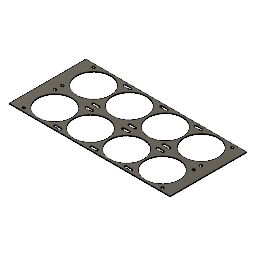
Corsair_1000D_120mm_x_8_fantray_extruded_v0 (Autodesk Fusion 360 design; units mm, degrees)
Autodesk Fusion 360 part; units mm, degrees
sketch "Sketch1" plane through (0, 0, 0) normal (0, 0, 1) x (1, 0, 0)
  line L0 (0, 0) -> (540, 0)
  line L1 (540, 0) -> (540, 258.064)
  line L2 (540, 258.064) -> (0, 258.064)
  line L3 (0, 258.064) -> (0, 0)
  circle A0 centre (89.662, 194.056) radius 56.642
  circle A1 centre (209.446, 194.056) radius 56.642
  line L4 (270, 258.064) -> (270, 0)
  line L5 (0, 129.032) -> (540, 129.032)
  circle A2 centre (450.3379, 194.056) radius 56.642
  circle A3 centre (330.5539, 194.056) radius 56.642
  circle A4 centre (89.662, 64.008) radius 56.642
  circle A5 centre (209.446, 64.008) radius 56.642
  circle A6 centre (330.5539, 64.008) radius 56.642
  circle A7 centre (450.3379, 64.008) radius 56.642
  line L6 (35.814, 249.428) -> (39.37, 249.428)
  line L7 (41.91, 246.888) -> (41.91, 245.11)
  line L8 (39.37, 242.57) -> (35.814, 242.57)
  line L9 (33.274, 245.11) -> (33.274, 246.888)
  arc A8 (35.814, 249.428) -> (33.274, 246.888) centre (35.814, 246.888) ccw
  arc A9 (33.274, 245.11) -> (35.814, 242.57) centre (35.814, 245.11) ccw
  arc A10 (39.37, 242.57) -> (41.91, 245.11) centre (39.37, 245.11) ccw
  arc A11 (41.91, 246.888) -> (39.37, 249.428) centre (39.37, 246.888) ccw
  line L10 (33.274, 140.208) -> (33.274, 141.986)
  arc A12 (33.274, 140.208) -> (35.814, 137.668) centre (35.814, 140.208) ccw
  line L11 (35.814, 144.526) -> (39.37, 144.526)
  arc A13 (35.814, 144.526) -> (33.274, 141.986) centre (35.814, 141.986) ccw
  line L12 (39.37, 137.668) -> (35.814, 137.668)
  line L13 (41.91, 141.986) -> (41.91, 140.208)
  arc A14 (39.37, 137.668) -> (41.91, 140.208) centre (39.37, 140.208) ccw
  arc A15 (41.91, 141.986) -> (39.37, 144.526) centre (39.37, 141.986) ccw
  line L14 (500.6299, 242.57) -> (504.1859, 242.57)
  line L15 (498.0899, 246.888) -> (498.0899, 245.11)
  arc A16 (506.7259, 246.888) -> (504.1859, 249.428) centre (504.1859, 246.888) ccw
  arc A17 (504.1859, 242.57) -> (506.7259, 245.11) centre (504.1859, 245.11) ccw
  arc A18 (498.0899, 245.11) -> (500.6299, 242.57) centre (500.6299, 245.11) ccw
  arc A19 (500.6299, 249.428) -> (498.0899, 246.888) centre (500.6299, 246.888) ccw
  line L16 (504.1859, 249.428) -> (500.6299, 249.428)
  line L17 (506.7259, 245.11) -> (506.7259, 246.888)
  arc A20 (39.37, 8.636) -> (41.91, 11.176) centre (39.37, 11.176) ccw
  arc A21 (35.814, 15.494) -> (33.274, 12.954) centre (35.814, 12.954) ccw
  line L18 (39.37, 15.494) -> (35.814, 15.494)
  arc A22 (33.274, 11.176) -> (35.814, 8.636) centre (35.814, 11.176) ccw
  line L19 (35.814, 8.636) -> (39.37, 8.636)
  line L20 (41.91, 11.176) -> (41.91, 12.954)
  arc A23 (41.91, 12.954) -> (39.37, 15.494) centre (39.37, 12.954) ccw
  line L21 (33.274, 12.954) -> (33.274, 11.176)
  arc A24 (35.814, 120.396) -> (33.274, 117.856) centre (35.814, 117.856) ccw
  line L22 (39.37, 120.396) -> (35.814, 120.396)
  line L23 (35.814, 113.538) -> (39.37, 113.538)
  line L24 (33.274, 117.856) -> (33.274, 116.078)
  arc A25 (39.37, 113.538) -> (41.91, 116.078) centre (39.37, 116.078) ccw
  arc A26 (33.274, 116.078) -> (35.814, 113.538) centre (35.814, 116.078) ccw
  arc A27 (41.91, 117.856) -> (39.37, 120.396) centre (39.37, 117.856) ccw
  line L25 (41.91, 116.078) -> (41.91, 117.856)
  line L26 (141.224, 249.428) -> (161.544, 249.428)
  line L27 (164.084, 246.888) -> (164.084, 245.11)
  line L28 (161.544, 242.57) -> (141.224, 242.57)
  line L29 (138.684, 245.11) -> (138.684, 246.888)
  arc A28 (138.684, 245.11) -> (141.224, 242.57) centre (141.224, 245.11) ccw
  arc A29 (141.224, 249.428) -> (138.684, 246.888) centre (141.224, 246.888) ccw
  arc A30 (161.544, 242.57) -> (164.084, 245.11) centre (161.544, 245.11) ccw
  arc A31 (164.084, 246.888) -> (161.544, 249.428) centre (161.544, 246.888) ccw
  line L30 (283.944, 242.57) -> (263.624, 242.57)
  line L31 (261.084, 245.11) -> (261.084, 246.888)
  line L32 (263.624, 249.428) -> (283.944, 249.428)
  arc A32 (286.484, 246.888) -> (283.944, 249.428) centre (283.944, 246.888) ccw
  line L33 (286.484, 246.888) -> (286.484, 245.11)
  arc A33 (283.944, 242.57) -> (286.484, 245.11) centre (283.944, 245.11) ccw
  arc A34 (261.084, 245.11) -> (263.624, 242.57) centre (263.624, 245.11) ccw
  arc A35 (263.624, 249.428) -> (261.084, 246.888) centre (263.624, 246.888) ccw
  arc A36 (138.684, 245.11) -> (141.224, 242.57) centre (141.224, 245.11) ccw
  arc A37 (141.224, 249.428) -> (138.684, 246.888) centre (141.224, 246.888) ccw
  line L34 (164.084, 246.888) -> (164.084, 245.11)
  arc A38 (161.544, 242.57) -> (164.084, 245.11) centre (161.544, 245.11) ccw
  line L35 (138.684, 245.11) -> (138.684, 246.888)
  arc A39 (164.084, 246.888) -> (161.544, 249.428) centre (161.544, 246.888) ccw
  line L36 (141.224, 249.428) -> (161.544, 249.428)
  line L37 (161.544, 242.57) -> (141.224, 242.57)
  line L38 (138.684, 138.852) -> (138.684, 140.63)
  line L39 (164.084, 140.63) -> (164.084, 138.852)
  line L40 (141.224, 143.17) -> (161.544, 143.17)
  arc A40 (164.084, 140.63) -> (161.544, 143.17) centre (161.544, 140.63) ccw
  arc A41 (138.684, 138.852) -> (141.224, 136.312) centre (141.224, 138.852) ccw
  line L41 (161.544, 136.312) -> (141.224, 136.312)
  arc A42 (141.224, 143.17) -> (138.684, 140.63) centre (141.224, 140.63) ccw
  arc A43 (161.544, 136.312) -> (164.084, 138.852) centre (161.544, 138.852) ccw
  arc A44 (261.084, 138.852) -> (263.624, 136.312) centre (263.624, 138.852) ccw
  line L42 (261.084, 138.852) -> (261.084, 140.63)
  line L43 (283.944, 136.312) -> (263.624, 136.312)
  arc A45 (283.944, 136.312) -> (286.484, 138.852) centre (283.944, 138.852) ccw
  arc A46 (263.624, 143.17) -> (261.084, 140.63) centre (263.624, 140.63) ccw
  line L44 (286.484, 140.63) -> (286.484, 138.852)
  arc A47 (286.484, 140.63) -> (283.944, 143.17) centre (283.944, 140.63) ccw
  line L45 (263.624, 143.17) -> (283.944, 143.17)
  line L46 (378.4559, 136.312) -> (398.7759, 136.312)
  arc A48 (375.9159, 138.852) -> (378.4559, 136.312) centre (378.4559, 138.852) ccw
  arc A49 (378.4559, 143.17) -> (375.9159, 140.63) centre (378.4559, 140.63) ccw
  arc A50 (398.7759, 136.312) -> (401.3159, 138.852) centre (398.7759, 138.852) ccw
  line L47 (398.7759, 143.17) -> (378.4559, 143.17)
  arc A51 (401.3159, 140.63) -> (398.7759, 143.17) centre (398.7759, 140.63) ccw
  line L48 (375.9159, 140.63) -> (375.9159, 138.852)
  line L49 (401.3159, 138.852) -> (401.3159, 140.63)
  line L50 (375.9159, 246.888) -> (375.9159, 245.11)
  line L51 (401.3159, 245.11) -> (401.3159, 246.888)
  line L52 (378.4559, 242.57) -> (398.7759, 242.57)
  arc A52 (398.7759, 242.57) -> (401.3159, 245.11) centre (398.7759, 245.11) ccw
  line L53 (398.7759, 249.428) -> (378.4559, 249.428)
  arc A53 (375.9159, 245.11) -> (378.4559, 242.57) centre (378.4559, 245.11) ccw
  line L54 (375.9159, 246.888) -> (375.9159, 245.11)
  arc A54 (401.3159, 246.888) -> (398.7759, 249.428) centre (398.7759, 246.888) ccw
  arc A55 (378.4559, 249.428) -> (375.9159, 246.888) centre (378.4559, 246.888) ccw
  arc A56 (375.9159, 245.11) -> (378.4559, 242.57) centre (378.4559, 245.11) ccw
  arc A57 (378.4559, 249.428) -> (375.9159, 246.888) centre (378.4559, 246.888) ccw
  line L55 (378.4559, 242.57) -> (398.7759, 242.57)
  arc A58 (398.7759, 242.57) -> (401.3159, 245.11) centre (398.7759, 245.11) ccw
  arc A59 (401.3159, 246.888) -> (398.7759, 249.428) centre (398.7759, 246.888) ccw
  line L56 (398.7759, 249.428) -> (378.4559, 249.428)
  line L57 (401.3159, 245.11) -> (401.3159, 246.888)
  arc A60 (398.7759, 8.636) -> (401.3159, 11.176) centre (398.7759, 11.176) ccw
  arc A61 (375.9159, 11.176) -> (378.4559, 8.636) centre (378.4559, 11.176) ccw
  line L58 (401.3159, 12.954) -> (401.3159, 11.176)
  line L59 (398.7759, 8.636) -> (378.4559, 8.636)
  arc A62 (401.3159, 12.954) -> (398.7759, 15.494) centre (398.7759, 12.954) ccw
  arc A63 (378.4559, 15.494) -> (375.9159, 12.954) centre (378.4559, 12.954) ccw
  line L60 (401.3159, 12.954) -> (401.3159, 11.176)
  arc A64 (378.4559, 15.494) -> (375.9159, 12.954) centre (378.4559, 12.954) ccw
  line L61 (398.7759, 8.636) -> (378.4559, 8.636)
  line L62 (375.9159, 11.176) -> (375.9159, 12.954)
  line L63 (375.9159, 11.176) -> (375.9159, 12.954)
  arc A65 (401.3159, 12.954) -> (398.7759, 15.494) centre (398.7759, 12.954) ccw
  arc A66 (398.7759, 8.636) -> (401.3159, 11.176) centre (398.7759, 11.176) ccw
  arc A67 (375.9159, 11.176) -> (378.4559, 8.636) centre (378.4559, 11.176) ccw
  line L64 (378.4559, 15.494) -> (398.7759, 15.494)
  line L65 (378.4559, 15.494) -> (398.7759, 15.494)
  line L66 (401.3159, 119.212) -> (401.3159, 117.434)
  arc A68 (378.4559, 121.752) -> (375.9159, 119.212) centre (378.4559, 119.212) ccw
  line L67 (398.7759, 114.894) -> (378.4559, 114.894)
  arc A69 (398.7759, 114.894) -> (401.3159, 117.434) centre (398.7759, 117.434) ccw
  arc A70 (375.9159, 117.434) -> (378.4559, 114.894) centre (378.4559, 117.434) ccw
  line L68 (378.4559, 121.752) -> (398.7759, 121.752)
  arc A71 (401.3159, 119.212) -> (398.7759, 121.752) centre (398.7759, 119.212) ccw
  line L69 (375.9159, 117.434) -> (375.9159, 119.212)
  line L70 (141.224, 114.894) -> (161.544, 114.894)
  arc A72 (161.544, 114.894) -> (164.084, 117.434) centre (161.544, 117.434) ccw
  line L71 (138.684, 119.212) -> (138.684, 117.434)
  arc A73 (141.224, 121.752) -> (138.684, 119.212) centre (141.224, 119.212) ccw
  arc A74 (164.084, 119.212) -> (161.544, 121.752) centre (161.544, 119.212) ccw
  line L72 (161.544, 121.752) -> (141.224, 121.752)
  arc A75 (138.684, 117.434) -> (141.224, 114.894) centre (141.224, 117.434) ccw
  line L73 (164.084, 117.434) -> (164.084, 119.212)
  line L74 (141.224, 8.636) -> (161.544, 8.636)
  line L75 (141.224, 8.636) -> (161.544, 8.636)
  line L76 (161.544, 15.494) -> (141.224, 15.494)
  line L77 (138.684, 12.954) -> (138.684, 11.176)
  line L78 (138.684, 12.954) -> (138.684, 11.176)
  line L79 (164.084, 11.176) -> (164.084, 12.954)
  arc A76 (141.224, 15.494) -> (138.684, 12.954) centre (141.224, 12.954) ccw
  arc A77 (161.544, 8.636) -> (164.084, 11.176) centre (161.544, 11.176) ccw
  arc A78 (161.544, 8.636) -> (164.084, 11.176) centre (161.544, 11.176) ccw
  arc A79 (138.684, 11.176) -> (141.224, 8.636) centre (141.224, 11.176) ccw
  line L80 (161.544, 15.494) -> (141.224, 15.494)
  arc A80 (141.224, 15.494) -> (138.684, 12.954) centre (141.224, 12.954) ccw
  arc A81 (164.084, 12.954) -> (161.544, 15.494) centre (161.544, 12.954) ccw
  line L81 (164.084, 11.176) -> (164.084, 12.954)
  arc A82 (164.084, 12.954) -> (161.544, 15.494) centre (161.544, 12.954) ccw
  arc A83 (138.684, 11.176) -> (141.224, 8.636) centre (141.224, 11.176) ccw
  arc A84 (286.484, 119.212) -> (283.944, 121.752) centre (283.944, 119.212) ccw
  arc A85 (263.624, 121.752) -> (261.084, 119.212) centre (263.624, 119.212) ccw
  line L82 (263.624, 114.894) -> (283.944, 114.894)
  arc A86 (283.944, 114.894) -> (286.484, 117.434) centre (283.944, 117.434) ccw
  line L83 (286.484, 117.434) -> (286.484, 119.212)
  line L84 (261.084, 119.212) -> (261.084, 117.434)
  line L85 (283.944, 121.752) -> (263.624, 121.752)
  arc A87 (261.084, 117.434) -> (263.624, 114.894) centre (263.624, 117.434) ccw
  arc A88 (261.084, 11.176) -> (263.624, 8.636) centre (263.624, 11.176) ccw
  arc A89 (283.944, 8.636) -> (286.484, 11.176) centre (283.944, 11.176) ccw
  arc A90 (286.484, 12.954) -> (283.944, 15.494) centre (283.944, 12.954) ccw
  arc A91 (263.624, 15.494) -> (261.084, 12.954) centre (263.624, 12.954) ccw
  line L86 (286.484, 11.176) -> (286.484, 12.954)
  line L87 (283.944, 15.494) -> (263.624, 15.494)
  line L88 (263.624, 8.636) -> (283.944, 8.636)
  line L89 (261.084, 12.954) -> (261.084, 11.176)
  arc A92 (504.1859, 137.668) -> (506.7259, 140.208) centre (504.1859, 140.208) ccw
  line L90 (506.7259, 140.208) -> (506.7259, 141.986)
  arc A93 (498.0899, 140.208) -> (500.6299, 137.668) centre (500.6299, 140.208) ccw
  line L91 (498.0899, 141.986) -> (498.0899, 140.208)
  arc A94 (506.7259, 141.986) -> (504.1859, 144.526) centre (504.1859, 141.986) ccw
  arc A95 (500.6299, 144.526) -> (498.0899, 141.986) centre (500.6299, 141.986) ccw
  line L92 (504.1859, 144.526) -> (500.6299, 144.526)
  line L93 (500.6299, 137.668) -> (504.1859, 137.668)
  line L94 (504.1859, 113.538) -> (500.6299, 113.538)
  arc A96 (504.1859, 113.538) -> (506.7259, 116.078) centre (504.1859, 116.078) ccw
  arc A97 (498.0899, 116.078) -> (500.6299, 113.538) centre (500.6299, 116.078) ccw
  line L95 (500.6299, 120.396) -> (504.1859, 120.396)
  line L96 (498.0899, 116.078) -> (498.0899, 117.856)
  arc A98 (506.7259, 117.856) -> (504.1859, 120.396) centre (504.1859, 117.856) ccw
  arc A99 (500.6299, 120.396) -> (498.0899, 117.856) centre (500.6299, 117.856) ccw
  line L97 (506.7259, 117.856) -> (506.7259, 116.078)
  line L98 (498.0899, 11.176) -> (498.0899, 12.954)
  arc A100 (500.6299, 15.494) -> (498.0899, 12.954) centre (500.6299, 12.954) ccw
  line L99 (500.6299, 15.494) -> (504.1859, 15.494)
  line L100 (506.7259, 12.954) -> (506.7259, 11.176)
  arc A101 (498.0899, 11.176) -> (500.6299, 8.636) centre (500.6299, 11.176) ccw
  line L101 (504.1859, 8.636) -> (500.6299, 8.636)
  arc A102 (504.1859, 8.636) -> (506.7259, 11.176) centre (504.1859, 11.176) ccw
  arc A103 (506.7259, 12.954) -> (504.1859, 15.494) centre (504.1859, 12.954) ccw
  point P0 (164.084, 249.428)
  point P1 (164.084, 242.57)
  point P2 (138.684, 242.57)
  point P3 (286.484, 249.428)
  point P4 (261.084, 242.57)
  point P5 (286.484, 242.57)
  point P6 (164.084, 249.428)
  point P7 (138.684, 242.57)
  point P8 (164.084, 242.57)
  point P9 (164.084, 143.17)
  point P10 (138.684, 136.312)
  point P11 (164.084, 136.312)
  point P12 (164.084, 146.05)
  point P13 (138.684, 146.05)
  point P14 (286.484, 136.312)
  point P15 (261.084, 136.312)
  point P16 (286.484, 143.17)
  point P17 (375.9159, 146.05)
  point P18 (401.3159, 136.312)
  point P19 (401.3159, 146.05)
  point P20 (375.9159, 143.17)
  point P21 (375.9159, 136.312)
  point P22 (375.9159, 242.57)
  point P23 (375.9159, 249.428)
  point P24 (375.9159, 242.57)
  point P25 (375.9159, 249.428)
  point P26 (401.3159, 242.57)
  point P27 (401.3159, 242.57)
  point P28 (375.9159, 15.494)
  point P29 (401.3159, 15.494)
  point P30 (375.9159, 8.636)
  point P31 (401.3159, 15.494)
  point P32 (375.9159, 8.636)
  point P33 (375.9159, 15.494)
  point P34 (401.3159, 121.752)
  point P35 (401.3159, 112.014)
  point P36 (375.9159, 114.894)
  point P37 (375.9159, 121.752)
  point P38 (375.9159, 112.014)
  point P39 (138.684, 112.014)
  point P40 (164.084, 121.752)
  point P41 (138.684, 121.752)
  point P42 (164.084, 114.894)
  point P43 (164.084, 112.014)
  point P44 (164.084, 8.636)
  point P45 (138.684, 15.494)
  point P46 (138.684, 15.494)
  point P47 (164.084, 15.494)
  point P48 (164.084, 8.636)
  point P49 (164.084, 15.494)
  point P50 (261.084, 121.752)
  point P51 (286.484, 114.894)
  point P52 (286.484, 121.752)
  point P53 (286.484, 15.494)
  point P54 (261.084, 15.494)
  point P55 (286.484, 8.636)
  dimension "d1" = 540
  dimension "d2" = 258.064
  dimension "d5" = 113.284
  dimension "d6" = 7.366
  dimension "d7" = 33.02
  dimension "d17" = 113.284
  dimension "d18" = 7.366
  dimension "d19" = 6.5
  dimension "d20" = 270
  dimension "d21" = 129.032
  dimension "d23" = 8.636
  dimension "d24" = 6.858
  dimension "d25" = 2.54
  dimension "d26" = 2.54
  dimension "d27" = 2.54
  dimension "d28" = 2.54
  dimension "d29" = 8.636
  dimension "d30" = 33.274
  dimension "d31" = 8.636
  dimension "d32" = 6.858
  dimension "d33" = 2.54
  dimension "d34" = 2.54
  dimension "d35" = 2.54
  dimension "d36" = 2.54
  dimension "d37" = 8.636
  dimension "d38" = 33.274
  dimension "d39" = 25.4
  dimension "d40" = 6.858
  dimension "d41" = 2.54
  dimension "d42" = 2.54
  dimension "d43" = 2.54
  dimension "d44" = 2.54
  dimension "d45" = 8.636
  dimension "d46" = 96.774
  dimension "d47" = 25.4
  dimension "d48" = 6.858
  dimension "d49" = 2.54
  dimension "d50" = 2.54
  dimension "d51" = 2.54
  dimension "d52" = 2.54
  dimension "d53" = 97
  dimension "d54" = 25.4
  dimension "d55" = 6.858
  dimension "d56" = 2.54
  dimension "d57" = 2.54
  dimension "d58" = 2.54
  dimension "d59" = 2.54
  dimension "d60" = 25.4
  dimension "d61" = 6.858
  dimension "d62" = 2.54
  dimension "d63" = 2.54
  dimension "d64" = 2.54
  dimension "d65" = 2.54
  dimension "d66" = 25.4
  dimension "d72" = 99.4
  dimension "d73" = 25.4
  dimension "d74" = 6.858
  dimension "d75" = 2.54
  dimension "d76" = 2.54
  dimension "d77" = 2.54
  dimension "d78" = 2.54
  dimension "d79" = 99.4
  constraint perpendicular L0 L1
  constraint parallel L0 L2
  constraint parallel L1 L3
  constraint horizontal L0
  constraint coincident L0.start L3.end
  constraint coincident L2 L4.start
  constraint coincident L0 L4.end
  constraint perpendicular L0 L4
  constraint coincident L3 L5.start
  constraint coincident L1 L5.end
  constraint perpendicular L1 L5
  constraint symmetric A0 L4 A2
  constraint symmetric A1 L4 A3
  constraint symmetric A0 L5 A4
  constraint symmetric A1 L5 A5
  constraint symmetric L5 A2 A7
  constraint symmetric L5 A3 A6
  constraint horizontal L6
  constraint vertical L7
  constraint horizontal L8
  constraint vertical L9
  constraint tangent L6 A8
  constraint tangent L9 A8
  constraint tangent L9 A9
  constraint tangent L8 A9
  constraint tangent L8 A10
  constraint tangent L7 A10
  constraint tangent L7 A11
  constraint tangent L6 A11
  constraint horizontal L11
  constraint vertical L13
  constraint horizontal L12
  constraint vertical L10
  constraint tangent L11 A13
  constraint tangent L10 A13
  constraint tangent L10 A12
  constraint tangent A12 L12
  constraint tangent L12 A14
  constraint tangent L13 A14
  constraint tangent L13 A15
  constraint tangent L11 A15
  constraint symmetric L4 L6.start A16.end
  constraint symmetric L4 L9.end A16.start
  constraint symmetric L4 A8 A16
  constraint symmetric L4 L9.start A17.end
  constraint symmetric L4 L8.end L14.end
  constraint symmetric L4 A9 A17
  constraint symmetric L4 L8.start L14.start
  constraint symmetric L4 L7.end L15.end
  constraint symmetric L4 A10 A18
  constraint symmetric L4 L7.start L15.start
  constraint symmetric L4 L6.end A19.start
  constraint symmetric L4 A11 A19
  constraint symmetric L5 L6.start A22.end
  constraint symmetric L5 L9.end A22.start
  constraint symmetric L5 A8 A22
  constraint symmetric L5 L9.start A21.end
  constraint symmetric L5 L8.end A21.start
  constraint symmetric L5 A9 A21
  constraint symmetric L5 L8.start L18.start
  constraint symmetric L5 L7.end L20.end
  constraint symmetric L5 A10 A23
  constraint symmetric L5 L7.start A20.end
  constraint symmetric L5 L6.end A20.start
  constraint symmetric L5 A11 A20
  constraint symmetric L5 L12.start L22.start
  constraint symmetric L5 L13.end A27.start
  constraint symmetric L5 L11.start L23.start
  constraint symmetric L5 L10.end L24.end
  constraint symmetric L5 L13.start A25.end
  constraint symmetric L5 L11.end L23.end
  constraint symmetric L5 L10.start A24.end
  constraint symmetric L5 A12.end A24.start
  constraint symmetric L5 A12 A24
  constraint symmetric L5 A13 A26
  constraint symmetric L5 A14 A27
  constraint symmetric L5 A15 A25
  constraint horizontal L26
  constraint vertical L27
  constraint horizontal L28
  constraint vertical L29
  constraint coincident P7 L28
  constraint coincident P7 L29
  constraint tangent L28 A28
  constraint tangent L29 A28
  constraint tangent L26 A29
  constraint tangent L29 A29
  constraint coincident P8 L28
  constraint coincident P8 L27
  constraint tangent L28 A30
  constraint tangent L27 A30
  constraint coincident P6 L26
  constraint coincident P6 L27
  constraint tangent L26 A31
  constraint tangent L27 A31
  constraint horizontal L32
  constraint vertical L33
  constraint horizontal L30
  constraint vertical L31
  constraint coincident P4 L30
  constraint coincident P4 L31
  constraint tangent L30 A34
  constraint tangent L31 A34
  constraint tangent L32 A35
  constraint tangent L31 A35
  constraint coincident P5 L30
  constraint coincident P5 L33
  constraint tangent L30 A33
  constraint tangent L33 A33
  constraint coincident P3 L32
  constraint coincident P3 L33
  constraint tangent L32 A32
  constraint tangent A32 L33
  constraint horizontal L36
  constraint vertical L34
  constraint horizontal L37
  constraint vertical L35
  constraint coincident P7 L37
  constraint coincident P7 L35
  constraint tangent A36 L37
  constraint tangent A36 L35
  constraint tangent A37 L36
  constraint tangent A37 L35
  constraint coincident P8 L37
  constraint coincident P8 L34
  constraint tangent A38 L37
  constraint tangent L34 A38
  constraint coincident P6 L36
  constraint coincident P6 L34
  constraint tangent A39 L36
  constraint tangent L34 A39
  constraint horizontal L40
  constraint vertical L39
  constraint horizontal L41
  constraint vertical L38
  constraint coincident P10 L41
  constraint coincident P10 L38
  constraint tangent A41 L41
  constraint tangent L38 A41
  constraint tangent L40 A42
  constraint tangent L38 A42
  constraint coincident P11 L41
  constraint coincident P11 L39
  constraint tangent L41 A43
  constraint tangent L39 A43
  constraint coincident P9 L40
  constraint coincident P9 L39
  constraint tangent L40 A40
  constraint tangent L39 A40
  constraint horizontal L45
  constraint vertical L44
  constraint horizontal L43
  constraint vertical L42
  constraint coincident P15 L43
  constraint coincident P15 L42
  constraint tangent A44 L43
  constraint tangent A44 L42
  constraint tangent A46 L45
  constraint tangent L42 A46
  constraint coincident P14 L43
  constraint coincident P14 L44
  constraint tangent L43 A45
  constraint tangent A45 L44
  constraint coincident P16 L45
  constraint coincident P16 L44
  constraint tangent A47 L45
  constraint tangent L44 A47
  constraint symmetric L4 P6 P25
  constraint symmetric L4 P8 P24
  constraint symmetric L4 P7 P27
  constraint symmetric L4 L28.end L52.end
  constraint symmetric L4 L29.start L51.start
  constraint symmetric L4 A28 A58
  constraint symmetric L4 L26.start L53.start
  constraint symmetric L4 L29.end L51.end
  constraint symmetric L4 A29 A59
  constraint symmetric L4 L28.start L52.start
  constraint symmetric L4 L27.end L50.end
  constraint symmetric L4 A30 A53
  constraint symmetric L4 L26.end L53.end
  constraint symmetric L4 L27.start L50.start
  constraint symmetric L4 A31 A57
  constraint symmetric L4 A36 A52
  constraint symmetric L4 A37 A54
  constraint symmetric L4 A38 A56
  constraint symmetric L4 A39 A55
  constraint symmetric L4 L39.start A49.end
  constraint symmetric L4 L40.end A49.start
  constraint symmetric L4 L40.start L47.start
  constraint symmetric L4 L38.end A51.start
  constraint symmetric L4 L41.start L46.start
  constraint symmetric L4 L39.end A48.start
  constraint symmetric L4 P9 P20
  constraint symmetric L4 P10 P18
  constraint symmetric L4 P11 P21
  constraint symmetric L4 A41.end L46.end
  constraint symmetric L4 L38.start A50.end
  constraint symmetric L4 P12 P17
  constraint symmetric L4 P13 P19
  constraint symmetric L4 A40 A49
  constraint symmetric L4 A41 A50
  constraint symmetric L4 A42 A51
  constraint symmetric L4 A43 A48
  constraint symmetric L5 P6 P48
  constraint symmetric L5 P8 P49
  constraint symmetric L5 P7 P46
  constraint symmetric L5 L28.end L76.end
  constraint symmetric L5 L29.start L77.start
  constraint symmetric L5 A28 A76
  constraint symmetric L5 L26.start L74.start
  constraint symmetric L5 L29.end L77.end
  constraint symmetric L5 A29 A83
  constraint symmetric L5 L28.start L76.start
  constraint symmetric L5 L27.end L79.end
  constraint symmetric L5 A30 A81
  constraint symmetric L5 L26.end L74.end
  constraint symmetric L5 L27.start L79.start
  constraint symmetric L5 A31 A78
  constraint symmetric L5 A32.start A89.end
  constraint symmetric L5 L32.end A89.start
  constraint symmetric L5 L32.start A88.end
  constraint symmetric L5 L31.end A88.start
  constraint symmetric L5 L30.start A90.end
  constraint symmetric L5 L33.end A90.start
  constraint symmetric L5 P3 P55
  constraint symmetric L5 P4 P54
  constraint symmetric L5 P5 P53
  constraint symmetric L5 L30.end A91.start
  constraint symmetric L5 L31.start A91.end
  constraint symmetric L5 A32 A89
  constraint symmetric L5 A33 A90
  constraint symmetric L5 A34 A91
  constraint symmetric L5 A35 A88
  constraint symmetric L5 A36 A80
  constraint symmetric L5 A37 A79
  constraint symmetric L5 A38 A82
  constraint symmetric L5 A39 A77
  constraint symmetric L5 L39.start A72.end
  constraint symmetric L5 L40.end L70.end
  constraint symmetric L5 L40.start L70.start
  constraint symmetric L5 L38.end L71.end
  constraint symmetric L5 L41.start A74.end
  constraint symmetric L5 L39.end A74.start
  constraint symmetric L5 P9 P42
  constraint symmetric L5 P10 P41
  constraint symmetric L5 P11 P40
  constraint symmetric L5 A41.end A73.start
  constraint symmetric L5 L38.start L71.start
  constraint symmetric L5 P12 P43
  constraint symmetric L5 P13 P39
  constraint symmetric L5 A40 A72
  constraint symmetric L5 A41 A73
  constraint symmetric L5 A42 A75
  constraint symmetric L5 A43 A74
  constraint symmetric L5 P14 P52
  constraint symmetric L5 P15 P50
  constraint symmetric L5 A44.start A85.end
  constraint symmetric L5 A44.end A85.start
  constraint symmetric L5 L44.start A86.end
  constraint symmetric L5 A47.end L82.end
  constraint symmetric L5 A46.start L82.start
  constraint symmetric L5 L42.end L84.end
  constraint symmetric L5 L43.start A84.end
  constraint symmetric L5 A45.end A84.start
  constraint symmetric L5 P16 P51
  constraint symmetric L5 A44 A85
  constraint symmetric L5 A45 A84
  constraint symmetric L5 A46 A87
  constraint symmetric L5 A47 A86
  constraint symmetric L5 L46.end L68.end
  constraint symmetric L5 A48.start A68.end
  constraint symmetric L5 P17 P38
  constraint symmetric L5 A49.start L67.end
  constraint symmetric L5 L47.start L67.start
  constraint symmetric L5 A51.start L66.end
  constraint symmetric L5 A50.end L66.start
  constraint symmetric L5 P18 P34
  constraint symmetric L5 P19 P35
  constraint symmetric L5 A49.end A70.start
  constraint symmetric L5 P20 P36
  constraint symmetric L5 P21 P37
  constraint symmetric L5 L46.start A68.start
  constraint symmetric L5 L51.end A60.end
  constraint symmetric L5 L53.start A60.start
  constraint symmetric L5 P24 P33
  constraint symmetric L5 P25 P32
  constraint symmetric L5 L53.end A61.end
  constraint symmetric L5 L51.start L58.start
  constraint symmetric L5 L50.start A61.start
  constraint symmetric L5 L52.end A62.end
  constraint symmetric L5 L50.end A63.end
  constraint symmetric L5 L52.start A63.start
  constraint symmetric L5 P27 P31
  constraint symmetric L5 A48 A68
  constraint symmetric L5 A49 A70
  constraint symmetric L5 A50 A71
  constraint symmetric L5 A51 A69
  constraint symmetric L5 A52 A65
  constraint symmetric L5 A53 A63
  constraint symmetric L5 A54 A60
  constraint symmetric L5 A55 A61
  constraint symmetric L5 A56 A64
  constraint symmetric L5 A57 A67
  constraint symmetric L5 A58 A62
  constraint symmetric L5 A59 A66
  constraint symmetric L4 L12.start A93.end
  constraint symmetric L4 L13.end A93.start
  constraint symmetric L4 L11.start A94.end
  constraint symmetric L4 L10.end L90.end
  constraint symmetric L4 L13.start L91.start
  constraint symmetric L4 L11.end A95.start
  constraint symmetric L4 L10.start A92.end
  constraint symmetric L4 A12.end A92.start
  constraint symmetric L4 A12 A92
  constraint symmetric L4 A13 A94
  constraint symmetric L4 A14 A93
  constraint symmetric L4 A15 A95
  constraint symmetric L5 A17.end L100.start
  constraint symmetric L5 L15.start L98.start
  constraint symmetric L5 A16.end L101.start
  constraint symmetric L5 L14.start A100.start
  constraint symmetric L5 A16.start L100.end
  constraint symmetric L5 A19.start A101.end
  constraint symmetric L5 L15.end L98.end
  constraint symmetric L5 L14.end L99.end
  constraint symmetric L5 A16 A102
  constraint symmetric L5 A17 A103
  constraint symmetric L5 A18 A100
  constraint symmetric L5 A19 A101
  constraint symmetric L5 A92.start L95.end
  constraint symmetric L5 A93.start L96.end
  constraint symmetric L5 L91.start A97.start
  constraint symmetric L5 A93.end L95.start
  constraint symmetric L5 A92.end A98.start
  constraint symmetric L5 A95.start L94.end
  constraint symmetric L5 A94.end L94.start
  constraint symmetric L5 L90.end A96.end
  constraint symmetric L5 A92 A98
  constraint symmetric L5 A93 A99
  constraint symmetric L5 A94 A96
  constraint symmetric L5 A95 A97
  measures "d1" distance of L0.start L0.end
  measures "d2" distance of L0.end L1.end
  measures "d5" diameter of A0
  measures "d6" distance of L2 A0
  measures "d7" distance of L3 A0
  measures "d17" diameter of A1
  measures "d18" distance of L2 A1
  measures "d19" distance of A0 A1
  measures "d20" distance of L3 L4
  measures "d21" distance of L2 L5
  measures "d23" distance of L7 L9
  measures "d24" distance of L6 L8
  measures "d25" radius of A8
  measures "d26" radius of A9
  measures "d27" radius of A10
  measures "d28" radius of A11
  measures "d29" distance of L2 L6
  measures "d30" distance of L3 L9
  measures "d31" distance of L10 L13
  measures "d32" distance of L11 L12
  measures "d33" radius of A13
  measures "d34" radius of A12
  measures "d35" radius of A14
  measures "d36" radius of A15
  measures "d37" distance of L5 L12
  measures "d38" distance of L3 L10
  measures "d39" distance of P8 P7
  measures "d40" distance of P6 P8
  measures "d41" radius of A28
  measures "d42" radius of A29
  measures "d43" radius of A30
  measures "d44" radius of A31
  measures "d45" distance of L2 L26
  measures "d46" distance of L7 L29
  measures "d47" distance of P4 P5
  measures "d48" distance of P3 P5
  measures "d49" radius of A34
  measures "d50" radius of A35
  measures "d51" radius of A33
  measures "d52" radius of A32
  measures "d53" distance of L27 L31
  measures "d54" distance of P7 P8
  measures "d55" distance of P6 P8
  measures "d56" radius of A36
  measures "d57" radius of A37
  measures "d58" radius of A38
  measures "d59" radius of A39
  measures "d60" distance of P10 P11
  measures "d61" distance of P9 P11
  measures "d62" radius of A41
  measures "d63" radius of A42
  measures "d64" radius of A43
  measures "d65" radius of A40
  measures "d66" distance of P12 P13
  measures "d72" distance of L28 L40
  measures "d73" distance of P14 P15
  measures "d74" distance of P14 P16
  measures "d75" radius of A44
  measures "d76" radius of A46
  measures "d77" radius of A45
  measures "d78" radius of A47
  measures "d79" distance of L30 L45
extrude "Extrude2" add sketch "Sketch1" along normal blind 2.54 contours L0 L3 L4 L5 A85 L82 L84 L85 A87 A88 A91 L87 L88 L89 | L0 L1 L4 L5 A84 L82 A86 L83 L85 A89 A90 L86 L87 L88 | L2 L3 L4 L5 L30 L31 L32 A34 A35 A44 L42 L43 A46 L45 | L1 L2 L4 L5 L30 L32 A32 L33 A33 L43 A45 L44 A47 L45
extrude "Extrude1" [suppressed]
